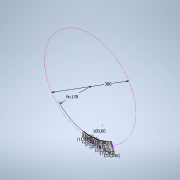
# Autodesk Inventor part: keywell_support-back
Saved by Autodesk Inventor 2020.1 (Build 241239000, 239)
## iProperties
Created: 2019-06-30
Part Number: keywell_support-back
Material: Acier inoxydable
Document SubType Name: Modeling
Designer: Thibault
Density: 8 g/cm^3
Appearance: Semi-poli
Mass: 13.686 g
Surface Area: 39.9351 cm^2
Volume: 1.71076 cm^3
kws_bp_anchor_dist1: 13,236 mm
kws_bp_anchor_dist2: 19,377 mm
kws_bp_anchor_dist3: 20,152 mm
kws_bp_anchor_dist4: 20,681 mm
kws_bp_anchor_dist5: 20,957 mm
kws_bp_anchor_dist6: 20,990 mm
kws_bp_anchor_dist7: 11,748 mm
Author: Thibault
Autodesk Inventor part; units mm, degrees
ref_plane "YZ Plane" through (0, 0, 0) normal (1, 0, 0) x (0, 1, 0)
ref_plane "XZ Plane" through (0, 0, 0) normal (0, 1, 0) x (-1, 0, 0)
ref_plane "XY Plane" through (0, 0, 0) normal (0, 0, 1) x (1, 0, 0)
sketch "Anchor (screw side)" plane through (0, 0, 0) normal (0, 0, 1) x (1, 0, 0)
  circle A0 centre (93.7216, 50.3096) radius 1.05
  line L0 (91.2716, 51.3596) -> (88.1716, 51.3596)
  line L1 (88.1716, 51.3596) -> (88.1716, 49.2596)
  line L2 (88.1716, 49.2596) -> (91.2716, 49.2596)
  line L3 (91.2716, 49.2596) -> (91.2716, 51.3596)
  line L4 (99.2716, 51.3596) -> (96.1716, 51.3596)
  line L5 (96.1716, 51.3596) -> (96.1716, 49.2596)
  line L6 (96.1716, 49.2596) -> (99.2716, 49.2596)
  line L7 (99.2716, 49.2596) -> (99.2716, 51.3596)
  line L8 (91.2716, 51.3596) -> (96.1716, 49.2596) construction
  line L9 (96.1716, 51.3596) -> (91.2716, 49.2596) construction
  line L10 (86.1716, 53.3596) -> (101.2716, 53.3596) construction
  line L11 (101.2716, 53.3596) -> (101.2716, 47.2596) construction
  line L12 (101.2716, 47.2596) -> (86.1716, 47.2596) construction
  line L13 (86.1716, 47.2596) -> (86.1716, 53.3596) construction
  point P0 (103.5798, 50.1132)
  dimension "d27" = 2.1
  dimension "d28" = 3.1
  dimension "d29" = 2.1
  dimension "d32_1" = 4.9
  dimension "d34" = 2
  dimension "d35" = 2
  dimension "d36" = 2
  dimension "d37" = 2
  measures "d27" diameter of A0
  measures "d28" distance of L2.end L1.end
  measures "d29" distance of L1.end L0.end
  measures "d32_1" distance between parallel lines of L5 L3
  measures "d34" distance between parallel lines of L0 L10
  measures "d35" distance between parallel lines of L12 L2
  measures "d36" distance between parallel lines of L11 L7
  measures "d37" distance between parallel lines of L13 L1
sketch "Anchor (nut side)" plane through (0, 0, 0) normal (0, 0, 1) x (1, 0, 0)
  line L0 (10, 0) -> (8.55, 0)
  line L1 (8.55, 0) -> (8.55, -2)
  line L2 (8.55, -2) -> (9.35, -2)
  line L3 (9.35, -2) -> (9.35, -4)
  line L4 (5.65, -4) -> (5.65, -2)
  line L5 (5.65, -2) -> (6.45, -2)
  line L6 (6.45, -2) -> (6.45, 0)
  line L7 (6.45, 0) -> (5, 0)
  line L8 (2, 0) -> (2, 2)
  line L9 (2, 0) -> (3, 0) construction
  line L10 (2, 2) -> (5, 2)
  line L11 (5, 2) -> (5, 0)
  line L12 (10, 0) -> (10, 2)
  line L13 (10, 2) -> (13, 2)
  line L14 (13, 2) -> (13, 0)
  line L15 (0, 0) -> (2, 0)
  line L16 (13, 0) -> (15, 0)
  line L17 (5.65, -4) -> (6.45, -4)
  line L18 (9.35, -4) -> (8.55, -4)
  line L19 (6.45, -4) -> (6.45, -6.25)
  line L20 (8.55, -4) -> (8.55, -6.25)
  line L21 (6.7, -6.5) -> (7.5, -6.5)
  arc A0 (6.45, -6.25) -> (6.7, -6.5) centre (6.7, -6.25) ccw
  arc A1 (8.3, -6.5) -> (8.55, -6.25) centre (8.3, -6.25) ccw
  line L22 (7.5, -6.5) -> (8.3, -6.5)
  line L23 (7.5, -3.8983) -> (7.5, -9.959) construction
  point P0 (9.1321, -0.6227)
  point P1 (6.45, -6.5)
  point P2 (8.55, -6.5)
  dimension "d3" = 2
  dimension "d7" = 5
  dimension "d10" = 1.45
  dimension "d11" = 2
  dimension "d12" = 0.8
  dimension "d13" = 2
  dimension "d14" = 0.8
  dimension "d15" = 2.1
  dimension "d18" = 2
  dimension "d19" = 0.8
  dimension "d20" = 0.8
  dimension "d21" = 2.5
  dimension "d22" = 2.5
  dimension "d23" = 2.1
  dimension "d38" = 2
  dimension "d39" = 0.25
  dimension "d120" = 3
  measures "d3" distance of point (0, 0) L8.start
  measures "d7" distance of L7.end L0.start
  measures "d10" distance of L0.start L0.end
  measures "d11" distance of L0.end L1.end
  measures "d12" distance of L1.end L2.end
  measures "d13" distance of L2.end L3.end
  measures "d14" distance of L4.end L5.end
  measures "d15" distance of L6.end L0.end
  measures "d18" distance of L14.end point (15, 0)
  measures "d19" distance of L4.start L17.end
  measures "d20" distance of L3.end L18.end
  measures "d21" distance of L17.end point (6.45, -6.5)
  measures "d22" distance of L18.end point (8.55, -6.5)
  measures "d23" distance of L17.end L18.end
  measures "d38" distance of the line from the sketch origin of L10
  measures "d39" radius of A0
  measures "d120" distance of L8.end L10.end
sketch "Screwless anchor (male)" plane through (0, 0, 0) normal (0, 0, 1) x (1, 0, 0)
  line L0 (2, 0) -> (2, 2)
  line L1 (2, 0) -> (3, 0) construction
  line L2 (2, 2) -> (5, 2)
  line L3 (5, 2) -> (5, 0)
  line L4 (10, 0) -> (10, 2)
  line L5 (10, 2) -> (13, 2)
  line L6 (13, 2) -> (13, 0)
  line L7 (0, 0) -> (2, 0)
  line L8 (13, 0) -> (15, 0)
  line L9 (5, 0) -> (10, 0)
  point P0 (9.1321, -0.6227)
  dimension "d81" = 2
  dimension "d83" = 5
  dimension "d92" = 2
  dimension "d100" = 2
  dimension "d119" = 3
  measures "d81" distance of L7.start L0.start
  measures "d83" distance of L3.end L4.start
  measures "d92" distance of L6.end L8.end
  measures "d100" distance between parallel lines of L7 L2
  measures "d119" distance of L0.end L2.end
sketch "Screwless anchor (female)" plane through (0, 0, 0) normal (0, 0, 1) x (1, 0, 0)
  line L0 (91.7814, 51.7592) -> (88.6814, 51.7592)
  line L1 (88.6814, 51.7592) -> (88.6814, 49.6592)
  line L2 (88.6814, 49.6592) -> (91.7814, 49.6592)
  line L3 (91.7814, 49.6592) -> (91.7814, 51.7592)
  line L4 (99.7814, 51.7592) -> (96.6814, 51.7592)
  line L5 (96.6814, 51.7592) -> (96.6814, 49.6592)
  line L6 (96.6814, 49.6592) -> (99.7814, 49.6592)
  line L7 (99.7814, 49.6592) -> (99.7814, 51.7592)
  line L8 (86.6814, 53.7592) -> (101.7814, 53.7592) construction
  line L9 (101.7814, 53.7592) -> (101.7814, 47.6592) construction
  line L10 (101.7814, 47.6592) -> (86.6814, 47.6592) construction
  line L11 (86.6814, 47.6592) -> (86.6814, 53.7592) construction
  point P0 (103.5798, 50.1132)
  dimension "d106" = 3.1
  dimension "d107" = 2.1
  dimension "d108" = 3.1
  dimension "d109" = 4.9
  dimension "d110" = 2
  dimension "d111" = 2
  dimension "d112" = 2
  dimension "d113" = 2
  measures "d106" distance of L2.end L1.end
  measures "d107" distance of L1.end L0.end
  measures "d108" distance of L6.end L5.end
  measures "d109" distance between parallel lines of L5 L3
  measures "d110" distance between parallel lines of L0 L8
  measures "d111" distance between parallel lines of L10 L2
  measures "d112" distance between parallel lines of L9 L7
  measures "d113" distance between parallel lines of L11 L1
sketch "Anchor" plane through (0, 0, 0) normal (0, 0, 1) x (1, 0, 0)
  line L0 (-55.5458, -124.6418) -> (-44.4458, -138.5418) construction
  line L1 (-44.4458, -124.6418) -> (-55.5458, -138.5418) construction
  line L2 (-49.9958, -129.7424) -> (-49.9958, -133.4154) construction
  circle A0 centre (-49.9958, -123.5918) radius 1.05
  line L3 (-52.4458, -122.5418) -> (-55.5458, -122.5418)
  line L4 (-55.5458, -122.5418) -> (-55.5458, -124.6418)
  line L5 (-55.5458, -124.6418) -> (-52.4458, -124.6418)
  line L6 (-52.4458, -124.6418) -> (-52.4458, -122.5418)
  line L7 (-44.4458, -122.5418) -> (-47.5458, -122.5418)
  line L8 (-47.5458, -122.5418) -> (-47.5458, -124.6418)
  line L9 (-47.5458, -124.6418) -> (-44.4458, -124.6418)
  line L10 (-44.4458, -124.6418) -> (-44.4458, -122.5418)
  line L11 (-52.4458, -122.5418) -> (-47.5458, -124.6418) construction
  line L12 (-47.5458, -122.5418) -> (-52.4458, -124.6418) construction
  line L13 (-57.5458, -120.5418) -> (-42.4458, -120.5418) construction
  line L14 (-42.4458, -120.5418) -> (-42.4458, -126.6418) construction
  line L15 (-42.4458, -126.6418) -> (-57.5458, -126.6418) construction
  line L16 (-57.5458, -126.6418) -> (-57.5458, -120.5418) construction
  circle A1 centre (-49.9958, -139.5918) radius 1.05
  line L17 (-52.4458, -138.5418) -> (-55.5458, -138.5418)
  line L18 (-55.5458, -138.5418) -> (-55.5458, -140.6418)
  line L19 (-55.5458, -140.6418) -> (-52.4458, -140.6418)
  line L20 (-52.4458, -140.6418) -> (-52.4458, -138.5418)
  line L21 (-44.4458, -138.5418) -> (-47.5458, -138.5418)
  line L22 (-47.5458, -138.5418) -> (-47.5458, -140.6418)
  line L23 (-47.5458, -140.6418) -> (-44.4458, -140.6418)
  line L24 (-44.4458, -140.6418) -> (-44.4458, -138.5418)
  line L25 (-52.4458, -138.5418) -> (-47.5458, -140.6418) construction
  line L26 (-47.5458, -138.5418) -> (-52.4458, -140.6418) construction
  line L27 (-57.5458, -136.5418) -> (-42.4458, -136.5418) construction
  line L28 (-42.4458, -136.5418) -> (-42.4458, -142.6418) construction
  line L29 (-42.4458, -142.6418) -> (-57.5458, -142.6418) construction
  line L30 (-57.5458, -142.6418) -> (-57.5458, -136.5418) construction
  point P0 (-66.8969, -206.6558)
  point P1 (-49.9958, -123.5918)
  dimension "d161" = 13.9
sketch "Esquisse2" plane through (0, 0, 0) normal (0, 0, 1) x (1, 0, 0)
  circle A0 centre (0, 0) radius 190 construction
  arc A1 (-29.0684, -175.6104) -> (87.3783, -155.0775) centre (0, 0) ccw
  line L0 (-31.0925, -195.4005) -> (-29.0684, -175.6104)
  line L1 (49.6599, -108.9569) -> (49.6599, -114.726) construction
  line L2 (96.0489, -172.9818) -> (96.0489, -198.8453)
  line L3 (-31.0925, -195.4005) -> (-31.0925, -198.8453)
  line L4 (30.9281, -182.0636) -> (33.2072, -181.6617) construction
  line L5 (87.3783, -155.0775) -> (96.0489, -172.9818)
  line L6 (-26.8444, -198.8453) -> (-31.0925, -198.8453)
  line L7 (-11.8444, -198.8453) -> (-5.8545, -198.8453)
  line L8 (9.1455, -198.8453) -> (15.1026, -198.8453)
  line L9 (30.1026, -198.8453) -> (35.7836, -198.8453)
  line L10 (50.7836, -198.8453) -> (55.9358, -198.8453)
  line L11 (70.9358, -198.8453) -> (75.313, -198.8453)
  line L12 (90.313, -198.8453) -> (96.0489, -198.8453)
  line L13 (28.843, -182.3134) -> (16.3622, -194.9882) construction
  line L14 (30.1635, -193.3346) -> (15.0417, -183.967) construction
  line L15 (24.4388, -188.4308) -> (20.7919, -188.8677) construction
  circle A2 centre (30.5458, -187.6991) radius 1.05
  line L16 (31.2969, -185.1416) -> (30.9281, -182.0636)
  line L17 (30.9281, -182.0636) -> (28.843, -182.3134)
  line L18 (28.843, -182.3134) -> (29.2118, -185.3914)
  line L19 (29.2118, -185.3914) -> (31.2969, -185.1416)
  line L20 (32.2486, -193.0848) -> (31.8798, -190.0068)
  line L21 (31.8798, -190.0068) -> (29.7947, -190.2566)
  line L22 (29.7947, -190.2566) -> (30.1635, -193.3346)
  line L23 (30.1635, -193.3346) -> (32.2486, -193.0848)
  line L24 (31.2969, -185.1416) -> (29.7947, -190.2566) construction
  line L25 (31.8798, -190.0068) -> (29.2118, -185.3914) construction
  line L26 (32.676, -179.8399) -> (34.4723, -194.8327) construction
  line L27 (34.4723, -194.8327) -> (28.4156, -195.5583) construction
  line L28 (28.4156, -195.5583) -> (26.6193, -180.5655) construction
  line L29 (26.6193, -180.5655) -> (32.676, -179.8399) construction
  circle A3 centre (14.6594, -189.6025) radius 1.05
  line L30 (15.4105, -187.045) -> (15.0417, -183.967)
  line L31 (15.0417, -183.967) -> (12.9566, -184.2168)
  line L32 (12.9566, -184.2168) -> (13.3254, -187.2948)
  line L33 (13.3254, -187.2948) -> (15.4105, -187.045)
  line L34 (16.3622, -194.9882) -> (15.9934, -191.9102)
  line L35 (15.9934, -191.9102) -> (13.9083, -192.16)
  line L36 (13.9083, -192.16) -> (14.2771, -195.238)
  line L37 (14.2771, -195.238) -> (16.3622, -194.9882)
  line L38 (15.4105, -187.045) -> (13.9083, -192.16) construction
  line L39 (15.9934, -191.9102) -> (13.3254, -187.2948) construction
  line L40 (16.7896, -181.7433) -> (18.5859, -196.736) construction
  line L41 (18.5859, -196.736) -> (12.5292, -197.4617) construction
  line L42 (12.5292, -197.4617) -> (10.7329, -182.4689) construction
  line L43 (10.7329, -182.4689) -> (16.7896, -181.7433) construction
  line L44 (86.6491, -162.9786) -> (78.9769, -179.0272) construction
  line L45 (91.4871, -172.9688) -> (74.1389, -169.0371) construction
  line L46 (84.4775, -170.1969) -> (81.1717, -171.7978) construction
  circle A4 centre (90.0132, -167.5161) radius 1.05
  line L47 (89.8903, -164.8534) -> (88.5392, -162.0633)
  line L48 (88.5392, -162.0633) -> (86.6491, -162.9786)
  line L49 (86.6491, -162.9786) -> (88.0003, -165.7687)
  line L50 (88.0003, -165.7687) -> (89.8903, -164.8534)
  line L51 (93.3772, -172.0535) -> (92.026, -169.2635)
  line L52 (92.026, -169.2635) -> (90.136, -170.1788)
  line L53 (90.136, -170.1788) -> (91.4871, -172.9688)
  line L54 (91.4871, -172.9688) -> (93.3772, -172.0535)
  line L55 (89.8903, -164.8534) -> (90.136, -170.1788) construction
  line L56 (92.026, -169.2635) -> (88.0003, -165.7687) construction
  line L57 (89.4675, -159.3916) -> (96.0489, -172.9818) construction
  line L58 (96.0489, -172.9818) -> (90.5588, -175.6405) construction
  line L59 (90.5588, -175.6405) -> (83.9774, -162.0503) construction
  line L60 (83.9774, -162.0503) -> (89.4675, -159.3916) construction
  circle A5 centre (75.6129, -174.4898) radius 1.05
  line L61 (75.4901, -171.8271) -> (74.1389, -169.0371)
  line L62 (74.1389, -169.0371) -> (72.2489, -169.9524)
  line L63 (72.2489, -169.9524) -> (73.6, -172.7424)
  line L64 (73.6, -172.7424) -> (75.4901, -171.8271)
  line L65 (78.9769, -179.0272) -> (77.6258, -176.2372)
  line L66 (77.6258, -176.2372) -> (75.7357, -177.1525)
  line L67 (75.7357, -177.1525) -> (77.0869, -179.9425)
  line L68 (77.0869, -179.9425) -> (78.9769, -179.0272)
  line L69 (75.4901, -171.8271) -> (75.7357, -177.1525) construction
  line L70 (77.6258, -176.2372) -> (73.6, -172.7424) construction
  line L71 (75.0672, -166.3653) -> (81.6487, -179.9555) construction
  line L72 (81.6487, -179.9555) -> (76.1586, -182.6143) construction
  line L73 (76.1586, -182.6143) -> (69.5771, -169.024) construction
  line L74 (69.5771, -169.024) -> (75.0672, -166.3653) construction
  line L75 (-5.2561, -195.6029) -> (8.5472, -184.3829) construction
  line L76 (-5.3523, -184.5033) -> (8.6433, -195.4825) construction
  line L77 (-0.2038, -190.0089) -> (3.4691, -189.9771) construction
  circle A6 centre (-6.3542, -190.0622) radius 1.05
  line L78 (-7.3829, -192.5212) -> (-7.3561, -195.621)
  line L79 (-7.3561, -195.621) -> (-5.2561, -195.6029)
  line L80 (-5.2561, -195.6029) -> (-5.283, -192.503)
  line L81 (-5.283, -192.503) -> (-7.3829, -192.5212)
  line L82 (-7.4522, -184.5215) -> (-7.4253, -187.6213)
  line L83 (-7.4253, -187.6213) -> (-5.3254, -187.6032)
  line L84 (-5.3254, -187.6032) -> (-5.3523, -184.5033)
  line L85 (-5.3523, -184.5033) -> (-7.4522, -184.5215)
  line L86 (-7.3829, -192.5212) -> (-5.3254, -187.6032) construction
  line L87 (-7.4253, -187.6213) -> (-5.283, -192.503) construction
  line L88 (-9.3387, -197.6383) -> (-9.4694, -182.5389) construction
  line L89 (-9.4694, -182.5389) -> (-3.3697, -182.486) construction
  line L90 (-3.3697, -182.486) -> (-3.2389, -197.5855) construction
  line L91 (-3.2389, -197.5855) -> (-9.3387, -197.6383) construction
  circle A7 centre (9.6452, -189.9236) radius 1.05
  line L92 (8.6165, -192.3826) -> (8.6433, -195.4825)
  line L93 (8.6433, -195.4825) -> (10.7433, -195.4643)
  line L94 (10.7433, -195.4643) -> (10.7164, -192.3644)
  line L95 (10.7164, -192.3644) -> (8.6165, -192.3826)
  line L96 (8.5472, -184.3829) -> (8.5741, -187.4828)
  line L97 (8.5741, -187.4828) -> (10.674, -187.4646)
  line L98 (10.674, -187.4646) -> (10.6471, -184.3647)
  line L99 (10.6471, -184.3647) -> (8.5472, -184.3829)
  line L100 (8.6165, -192.3826) -> (10.674, -187.4646) construction
  line L101 (8.5741, -187.4828) -> (10.7164, -192.3644) construction
  line L102 (6.6607, -197.4997) -> (6.53, -182.4003) construction
  line L103 (6.53, -182.4003) -> (12.6297, -182.3475) construction
  line L104 (12.6297, -182.3475) -> (12.7605, -197.4469) construction
  line L105 (12.7605, -197.4469) -> (6.6607, -197.4997) construction
  line L106 (-26.8103, -193.8281) -> (-11.853, -184.1999) construction
  line L107 (-25.6809, -182.7857) -> (-12.9824, -195.2423) construction
  line L108 (-21.1714, -188.8258) -> (-17.5175, -189.1995) construction
  circle A8 centre (-27.2901, -188.2) radius 1.05
  line L109 (-28.5839, -190.5305) -> (-28.8994, -193.6144)
  line L110 (-28.8994, -193.6144) -> (-26.8103, -193.8281)
  line L111 (-26.8103, -193.8281) -> (-26.4948, -190.7441)
  line L112 (-26.4948, -190.7441) -> (-28.5839, -190.5305)
  line L113 (-27.77, -182.572) -> (-28.0854, -185.6559)
  line L114 (-28.0854, -185.6559) -> (-25.9963, -185.8696)
  line L115 (-25.9963, -185.8696) -> (-25.6809, -182.7857)
  line L116 (-25.6809, -182.7857) -> (-27.77, -182.572)
  line L117 (-28.5839, -190.5305) -> (-25.9963, -185.8696) construction
  line L118 (-28.0854, -185.6559) -> (-26.4948, -190.7441) construction
  line L119 (-31.0925, -195.4005) -> (-29.5561, -180.3789) construction
  line L120 (-29.5561, -180.3789) -> (-23.4878, -180.9995) construction
  line L121 (-23.4878, -180.9995) -> (-25.0241, -196.0212) construction
  line L122 (-25.0241, -196.0212) -> (-31.0925, -195.4005) construction
  circle A9 centre (-11.3732, -189.828) radius 1.05
  line L123 (-12.667, -192.1584) -> (-12.9824, -195.2423)
  line L124 (-12.9824, -195.2423) -> (-10.8933, -195.456)
  line L125 (-10.8933, -195.456) -> (-10.5779, -192.3721)
  line L126 (-10.5779, -192.3721) -> (-12.667, -192.1584)
  line L127 (-11.853, -184.1999) -> (-12.1684, -187.2838)
  line L128 (-12.1684, -187.2838) -> (-10.0793, -187.4975)
  line L129 (-10.0793, -187.4975) -> (-9.7639, -184.4136)
  line L130 (-9.7639, -184.4136) -> (-11.853, -184.1999)
  line L131 (-12.667, -192.1584) -> (-10.0793, -187.4975) construction
  line L132 (-12.1684, -187.2838) -> (-10.5779, -192.3721) construction
  line L133 (-15.1755, -197.0284) -> (-13.6391, -182.0068) construction
  line L134 (-13.6391, -182.0068) -> (-7.5708, -182.6275) construction
  line L135 (-7.5708, -182.6275) -> (-9.1072, -197.6491) construction
  line L136 (-9.1072, -197.6491) -> (-15.1755, -197.0284) construction
  line L137 (48.7865, -178.0168) -> (37.7806, -191.9915) construction
  line L138 (51.3152, -188.8249) -> (35.252, -181.1833) construction
  line L139 (45.0843, -184.5828) -> (41.5079, -185.4196) construction
  circle A10 centre (51.0732, -183.1817) radius 1.05
  line L140 (51.5375, -180.5569) -> (50.8313, -177.5384)
  line L141 (50.8313, -177.5384) -> (48.7865, -178.0168)
  line L142 (48.7865, -178.0168) -> (49.4927, -181.0353)
  line L143 (49.4927, -181.0353) -> (51.5375, -180.5569)
  line L144 (53.3599, -188.3465) -> (52.6537, -185.3281)
  line L145 (52.6537, -185.3281) -> (50.6089, -185.8065)
  line L146 (50.6089, -185.8065) -> (51.3152, -188.8249)
  line L147 (51.3152, -188.8249) -> (53.3599, -188.3465)
  line L148 (51.5375, -180.5569) -> (50.6089, -185.8065) construction
  line L149 (52.6537, -185.3281) -> (49.4927, -181.0353) construction
  line L150 (52.3231, -175.1354) -> (55.763, -189.8383) construction
  line L151 (55.763, -189.8383) -> (49.8234, -191.228) construction
  line L152 (49.8234, -191.228) -> (46.3835, -176.525) construction
  line L153 (46.3835, -176.525) -> (52.3231, -175.1354) construction
  circle A11 centre (35.4939, -186.8266) radius 1.05
  line L154 (35.9582, -184.2018) -> (35.252, -181.1833)
  line L155 (35.252, -181.1833) -> (33.2072, -181.6617)
  line L156 (33.2072, -181.6617) -> (33.9134, -184.6802)
  line L157 (33.9134, -184.6802) -> (35.9582, -184.2018)
  line L158 (37.7806, -191.9915) -> (37.0744, -188.973)
  line L159 (37.0744, -188.973) -> (35.0297, -189.4514)
  line L160 (35.0297, -189.4514) -> (35.7359, -192.4699)
  line L161 (35.7359, -192.4699) -> (37.7806, -191.9915)
  line L162 (35.9582, -184.2018) -> (35.0297, -189.4514) construction
  line L163 (37.0744, -188.973) -> (33.9134, -184.6802) construction
  line L164 (36.7438, -178.7803) -> (40.1837, -193.4833) construction
  line L165 (40.1837, -193.4833) -> (34.2441, -194.8729) construction
  line L166 (34.2441, -194.8729) -> (30.8042, -180.1699) construction
  line L167 (30.8042, -180.1699) -> (36.7438, -178.7803) construction
  line L168 (68.134, -171.5455) -> (58.7376, -186.6494) construction
  line L169 (71.84, -182.0086) -> (55.0316, -176.1864) construction
  line L170 (65.179, -178.48) -> (61.7168, -179.7063) construction
  circle A12 centre (70.9767, -176.4265) radius 1.05
  line L171 (71.1485, -173.7665) -> (70.1135, -170.8444)
  line L172 (70.1135, -170.8444) -> (68.134, -171.5455)
  line L173 (68.134, -171.5455) -> (69.169, -174.4676)
  line L174 (69.169, -174.4676) -> (71.1485, -173.7665)
  line L175 (73.8194, -181.3075) -> (72.7844, -178.3853)
  line L176 (72.7844, -178.3853) -> (70.8049, -179.0865)
  line L177 (70.8049, -179.0865) -> (71.84, -182.0086)
  line L178 (71.84, -182.0086) -> (73.8194, -181.3075)
  line L179 (71.1485, -173.7665) -> (70.8049, -179.0865) construction
  line L180 (72.7844, -178.3853) -> (69.169, -174.4676) construction
  line L181 (71.331, -168.2914) -> (76.3724, -182.5249) construction
  line L182 (76.3724, -182.5249) -> (70.6225, -184.5616) construction
  line L183 (70.6225, -184.5616) -> (65.581, -170.328) construction
  line L184 (65.581, -170.328) -> (71.331, -168.2914) construction
  circle A13 centre (55.8948, -181.7685) radius 1.05
  line L185 (56.0666, -179.1085) -> (55.0316, -176.1864)
  line L186 (55.0316, -176.1864) -> (53.0521, -176.8875)
  line L187 (53.0521, -176.8875) -> (54.0871, -179.8096)
  line L188 (54.0871, -179.8096) -> (56.0666, -179.1085)
  line L189 (58.7376, -186.6494) -> (57.7026, -183.7273)
  line L190 (57.7026, -183.7273) -> (55.7231, -184.4284)
  line L191 (55.7231, -184.4284) -> (56.7581, -187.3505)
  line L192 (56.7581, -187.3505) -> (58.7376, -186.6494)
  line L193 (56.0666, -179.1085) -> (55.7231, -184.4284) construction
  line L194 (57.7026, -183.7273) -> (54.0871, -179.8096) construction
  line L195 (56.2491, -173.6334) -> (61.2905, -187.8669) construction
  line L196 (61.2905, -187.8669) -> (55.5406, -189.9035) construction
  line L197 (55.5406, -189.9035) -> (50.4991, -175.67) construction
  line L198 (50.4991, -175.67) -> (56.2491, -173.6334) construction
  line L199 (-21.8444, -198.8453) -> (-20.3944, -198.8453)
  line L200 (-20.3944, -198.8453) -> (-20.3944, -196.8453)
  line L201 (-20.3944, -196.8453) -> (-21.1944, -196.8453)
  line L202 (-21.1944, -196.8453) -> (-21.1944, -194.8453)
  line L203 (-17.4944, -194.8453) -> (-17.4944, -196.8453)
  line L204 (-17.4944, -196.8453) -> (-18.2944, -196.8453)
  line L205 (-18.2944, -196.8453) -> (-18.2944, -198.8453)
  line L206 (-18.2944, -198.8453) -> (-16.8444, -198.8453)
  line L207 (-13.8444, -198.8453) -> (-13.8444, -200.8453)
  line L208 (-13.8444, -198.8453) -> (-14.8444, -198.8453) construction
  line L209 (-13.8444, -200.8453) -> (-16.8444, -200.8453)
  line L210 (-16.8444, -200.8453) -> (-16.8444, -198.8453)
  line L211 (-21.8444, -198.8453) -> (-21.8444, -200.8453)
  line L212 (-21.8444, -200.8453) -> (-24.8444, -200.8453)
  line L213 (-24.8444, -200.8453) -> (-24.8444, -198.8453)
  line L214 (-11.8444, -198.8453) -> (-13.8444, -198.8453)
  line L215 (-24.8444, -198.8453) -> (-26.8444, -198.8453)
  line L216 (-17.4944, -194.8453) -> (-18.2944, -194.8453)
  line L217 (-21.1944, -194.8453) -> (-20.3944, -194.8453)
  line L218 (-18.2944, -194.8453) -> (-18.2944, -192.5953)
  line L219 (-20.3944, -194.8453) -> (-20.3944, -192.5953)
  line L220 (-18.5444, -192.3453) -> (-19.3444, -192.3453)
  arc A14 (-18.2944, -192.5953) -> (-18.5444, -192.3453) centre (-18.5444, -192.5953) ccw
  arc A15 (-20.1444, -192.3453) -> (-20.3944, -192.5953) centre (-20.1444, -192.5953) ccw
  line L221 (-19.3444, -192.3453) -> (-20.1444, -192.3453)
  line L222 (-19.3444, -194.9471) -> (-19.3444, -188.8863) construction
  line L223 (-0.8545, -198.8453) -> (0.5955, -198.8453)
  line L224 (0.5955, -198.8453) -> (0.5955, -196.8453)
  line L225 (0.5955, -196.8453) -> (-0.2045, -196.8453)
  line L226 (-0.2045, -196.8453) -> (-0.2045, -194.8453)
  line L227 (3.4955, -194.8453) -> (3.4955, -196.8453)
  line L228 (3.4955, -196.8453) -> (2.6955, -196.8453)
  line L229 (2.6955, -196.8453) -> (2.6955, -198.8453)
  line L230 (2.6955, -198.8453) -> (4.1455, -198.8453)
  line L231 (7.1455, -198.8453) -> (7.1455, -200.8453)
  line L232 (7.1455, -198.8453) -> (6.1455, -198.8453) construction
  line L233 (7.1455, -200.8453) -> (4.1455, -200.8453)
  line L234 (4.1455, -200.8453) -> (4.1455, -198.8453)
  line L235 (-0.8545, -198.8453) -> (-0.8545, -200.8453)
  line L236 (-0.8545, -200.8453) -> (-3.8545, -200.8453)
  line L237 (-3.8545, -200.8453) -> (-3.8545, -198.8453)
  line L238 (9.1455, -198.8453) -> (7.1455, -198.8453)
  line L239 (-3.8545, -198.8453) -> (-5.8545, -198.8453)
  line L240 (3.4955, -194.8453) -> (2.6955, -194.8453)
  line L241 (-0.2045, -194.8453) -> (0.5955, -194.8453)
  line L242 (2.6955, -194.8453) -> (2.6955, -192.5953)
  line L243 (0.5955, -194.8453) -> (0.5955, -192.5953)
  line L244 (2.4455, -192.3453) -> (1.6455, -192.3453)
  arc A16 (2.6955, -192.5953) -> (2.4455, -192.3453) centre (2.4455, -192.5953) ccw
  arc A17 (0.8455, -192.3453) -> (0.5955, -192.5953) centre (0.8455, -192.5953) ccw
  line L245 (1.6455, -192.3453) -> (0.8455, -192.3453)
  line L246 (1.6455, -194.9471) -> (1.6455, -188.8863) construction
  line L247 (20.1026, -198.8453) -> (21.5526, -198.8453)
  line L248 (21.5526, -198.8453) -> (21.5526, -196.8453)
  line L249 (21.5526, -196.8453) -> (20.7526, -196.8453)
  line L250 (20.7526, -196.8453) -> (20.7526, -194.8453)
  line L251 (24.4526, -194.8453) -> (24.4526, -196.8453)
  line L252 (24.4526, -196.8453) -> (23.6526, -196.8453)
  line L253 (23.6526, -196.8453) -> (23.6526, -198.8453)
  line L254 (23.6526, -198.8453) -> (25.1026, -198.8453)
  line L255 (28.1026, -198.8453) -> (28.1026, -200.8453)
  line L256 (28.1026, -198.8453) -> (27.1026, -198.8453) construction
  line L257 (28.1026, -200.8453) -> (25.1026, -200.8453)
  line L258 (25.1026, -200.8453) -> (25.1026, -198.8453)
  line L259 (20.1026, -198.8453) -> (20.1026, -200.8453)
  line L260 (20.1026, -200.8453) -> (17.1026, -200.8453)
  line L261 (17.1026, -200.8453) -> (17.1026, -198.8453)
  line L262 (30.1026, -198.8453) -> (28.1026, -198.8453)
  line L263 (17.1026, -198.8453) -> (15.1026, -198.8453)
  line L264 (24.4526, -194.8453) -> (23.6526, -194.8453)
  line L265 (20.7526, -194.8453) -> (21.5526, -194.8453)
  line L266 (23.6526, -194.8453) -> (23.6526, -192.5953)
  line L267 (21.5526, -194.8453) -> (21.5526, -192.5953)
  line L268 (23.4026, -192.3453) -> (22.6026, -192.3453)
  arc A18 (23.6526, -192.5953) -> (23.4026, -192.3453) centre (23.4026, -192.5953) ccw
  arc A19 (21.8026, -192.3453) -> (21.5526, -192.5953) centre (21.8026, -192.5953) ccw
  line L269 (22.6026, -192.3453) -> (21.8026, -192.3453)
  line L270 (22.6026, -194.9471) -> (22.6026, -188.8863) construction
  line L271 (40.7836, -198.8453) -> (42.2336, -198.8453)
  line L272 (42.2336, -198.8453) -> (42.2336, -196.8453)
  line L273 (42.2336, -196.8453) -> (41.4336, -196.8453)
  line L274 (41.4336, -196.8453) -> (41.4336, -194.8453)
  line L275 (45.1336, -194.8453) -> (45.1336, -196.8453)
  line L276 (45.1336, -196.8453) -> (44.3336, -196.8453)
  line L277 (44.3336, -196.8453) -> (44.3336, -198.8453)
  line L278 (44.3336, -198.8453) -> (45.7836, -198.8453)
  line L279 (48.7836, -198.8453) -> (48.7836, -200.8453)
  line L280 (48.7836, -198.8453) -> (47.7836, -198.8453) construction
  line L281 (48.7836, -200.8453) -> (45.7836, -200.8453)
  line L282 (45.7836, -200.8453) -> (45.7836, -198.8453)
  line L283 (40.7836, -198.8453) -> (40.7836, -200.8453)
  line L284 (40.7836, -200.8453) -> (37.7836, -200.8453)
  line L285 (37.7836, -200.8453) -> (37.7836, -198.8453)
  line L286 (50.7836, -198.8453) -> (48.7836, -198.8453)
  line L287 (37.7836, -198.8453) -> (35.7836, -198.8453)
  line L288 (45.1336, -194.8453) -> (44.3336, -194.8453)
  line L289 (41.4336, -194.8453) -> (42.2336, -194.8453)
  line L290 (44.3336, -194.8453) -> (44.3336, -192.5953)
  line L291 (42.2336, -194.8453) -> (42.2336, -192.5953)
  line L292 (44.0836, -192.3453) -> (43.2836, -192.3453)
  arc A20 (44.3336, -192.5953) -> (44.0836, -192.3453) centre (44.0836, -192.5953) ccw
  arc A21 (42.4836, -192.3453) -> (42.2336, -192.5953) centre (42.4836, -192.5953) ccw
  line L293 (43.2836, -192.3453) -> (42.4836, -192.3453)
  line L294 (43.2836, -194.9471) -> (43.2836, -188.8863) construction
  line L295 (60.9358, -198.8453) -> (62.3858, -198.8453)
  line L296 (62.3858, -198.8453) -> (62.3858, -196.8453)
  line L297 (62.3858, -196.8453) -> (61.5858, -196.8453)
  line L298 (61.5858, -196.8453) -> (61.5858, -194.8453)
  line L299 (65.2858, -194.8453) -> (65.2858, -196.8453)
  line L300 (65.2858, -196.8453) -> (64.4858, -196.8453)
  line L301 (64.4858, -196.8453) -> (64.4858, -198.8453)
  line L302 (64.4858, -198.8453) -> (65.9358, -198.8453)
  line L303 (68.9358, -198.8453) -> (68.9358, -200.8453)
  line L304 (68.9358, -198.8453) -> (67.9358, -198.8453) construction
  line L305 (68.9358, -200.8453) -> (65.9358, -200.8453)
  line L306 (65.9358, -200.8453) -> (65.9358, -198.8453)
  line L307 (60.9358, -198.8453) -> (60.9358, -200.8453)
  line L308 (60.9358, -200.8453) -> (57.9358, -200.8453)
  line L309 (57.9358, -200.8453) -> (57.9358, -198.8453)
  line L310 (70.9358, -198.8453) -> (68.9358, -198.8453)
  line L311 (57.9358, -198.8453) -> (55.9358, -198.8453)
  line L312 (65.2858, -194.8453) -> (64.4858, -194.8453)
  line L313 (61.5858, -194.8453) -> (62.3858, -194.8453)
  line L314 (64.4858, -194.8453) -> (64.4858, -192.5953)
  line L315 (62.3858, -194.8453) -> (62.3858, -192.5953)
  line L316 (64.2358, -192.3453) -> (63.4358, -192.3453)
  arc A22 (64.4858, -192.5953) -> (64.2358, -192.3453) centre (64.2358, -192.5953) ccw
  arc A23 (62.6358, -192.3453) -> (62.3858, -192.5953) centre (62.6358, -192.5953) ccw
  line L317 (63.4358, -192.3453) -> (62.6358, -192.3453)
  line L318 (63.4358, -194.9471) -> (63.4358, -188.8863) construction
  line L319 (80.313, -198.8453) -> (81.763, -198.8453)
  line L320 (81.763, -198.8453) -> (81.763, -196.8453)
  line L321 (81.763, -196.8453) -> (80.963, -196.8453)
  line L322 (80.963, -196.8453) -> (80.963, -194.8453)
  line L323 (84.663, -194.8453) -> (84.663, -196.8453)
  line L324 (84.663, -196.8453) -> (83.863, -196.8453)
  line L325 (83.863, -196.8453) -> (83.863, -198.8453)
  line L326 (83.863, -198.8453) -> (85.313, -198.8453)
  line L327 (88.313, -198.8453) -> (88.313, -200.8453)
  line L328 (88.313, -198.8453) -> (87.313, -198.8453) construction
  line L329 (88.313, -200.8453) -> (85.313, -200.8453)
  line L330 (85.313, -200.8453) -> (85.313, -198.8453)
  line L331 (80.313, -198.8453) -> (80.313, -200.8453)
  line L332 (80.313, -200.8453) -> (77.313, -200.8453)
  line L333 (77.313, -200.8453) -> (77.313, -198.8453)
  line L334 (90.313, -198.8453) -> (88.313, -198.8453)
  line L335 (77.313, -198.8453) -> (75.313, -198.8453)
  line L336 (84.663, -194.8453) -> (83.863, -194.8453)
  line L337 (80.963, -194.8453) -> (81.763, -194.8453)
  line L338 (83.863, -194.8453) -> (83.863, -192.5953)
  line L339 (81.763, -194.8453) -> (81.763, -192.5953)
  line L340 (83.613, -192.3453) -> (82.813, -192.3453)
  arc A24 (83.863, -192.5953) -> (83.613, -192.3453) centre (83.613, -192.5953) ccw
  arc A25 (82.013, -192.3453) -> (81.763, -192.5953) centre (82.013, -192.5953) ccw
  line L341 (82.813, -192.3453) -> (82.013, -192.3453)
  line L342 (82.813, -194.9471) -> (82.813, -188.8863) construction
  point P0 (1.6455, -189.9929)
  point P1 (-19.3316, -189.014)
  point P2 (43.2836, -185.0041)
  point P3 (63.4358, -179.0975)
  point P4 (22.6026, -188.6508)
  point P5 (82.813, -171.0029)
  point P6 (-19.3316, -189.014)
  point P7 (1.6455, -189.9929)
  point P8 (22.6026, -188.6508)
  point P9 (63.4358, -179.0975)
  point P10 (82.813, -171.0029)
  point P11 (82.813, -171.0029)
  point P12 (63.4358, -179.0975)
  point P13 (43.2836, -185.0041)
  point P14 (22.6026, -188.6508)
  point P15 (1.6455, -189.9929)
  point P16 (-19.3444, -189.0127)
  dimension "kws_bp_anchor_dist2" = 19.3773
  dimension "kws_bp_anchor_dist3" = 20.1522
  dimension "kws_bp_anchor_dist4" = 20.681
  dimension "kws_bp_anchor_dist5" = 20.9571
  dimension "kws_bp_anchor_dist6" = 20.99
  dimension "radius" = 380
  dimension "d73" = 178
  dimension "d163" = 21
  dimension "d164" = 21
  dimension "d165" = 21
  dimension "d166" = 21
  dimension "d167" = 21
  dimension "d170" = 80
  dimension "kws_bp_anchor_dist1" = 13.236
  dimension "kws_bp_anchor_dist7" = 11.748
  constraints: 26 end point, 8 point on circle, 7 horizontal, 3 vertical, 2 centre point, 1 coincident, 49 other
  measures "radius" diameter of A0
  measures "d73" radius of A1
  measures "d163" distance of A0.start A0.end
  measures "d164" distance of point (22.603, -188.651) point (43.284, -185.004)
  measures "d165" distance of point (43.284, -185.004) point (63.436, -179.097)
  measures "d166" distance of point (63.436, -179.097) point (82.813, -171.003)
  measures "d167" distance of A0.start point (22.603, -188.651)
  measures "d170" angle of L4 L1
extrude "Base" add sketch "Esquisse2" along normal blind 2
sketch "Esquisse5" plane through (0, 0, 2) normal (0, 0, 1) x (1, 0, 0)
  line L0 (50.2059, -108.6494) -> (185.6965, -108.6494)
  line L1 (185.6965, -108.6494) -> (185.6965, -257.0945)
  line L2 (50.2059, -108.6494) -> (76.3724, -182.5249)
  line L3 (76.3724, -182.5249) -> (76.3724, -257.0945)
  line L4 (76.3724, -257.0945) -> (185.6965, -257.0945)
  line L5 (70.1135, -170.8444) -> (71.1485, -173.7665) projected
  line L6 (73.8194, -181.3075) -> (71.84, -182.0086) projected
  point P0 (0, 0)
  dimension "d171" = 2
  dimension "d172" = 2
  constraints: 10 end point, 2 perpendicular, 1 horizontal, 1 parallel, 1 vertical
  measures "d171" distance between parallel lines of L5 L2
  measures "d172" distance from line of L2.end L6
extrude "Front: substract" [suppressed]
sketch "Esquisse7" plane through (0, 0, 2) normal (0, 0, 1) x (1, 0, 0)
  line L0 (74.4872, -183.1927) -> (56.3302, -131.9301)
  line L1 (72.7854, -178.388) -> (73.2029, -179.5666)
  line L2 (-107.1306, -265.4008) -> (-95.5548, -119.8506)
  line L3 (-95.5548, -119.8506) -> (56.3302, -131.9301)
  line L4 (74.4872, -183.1927) -> (74.4872, -265.4008)
  line L5 (74.4872, -265.4008) -> (-107.1306, -265.4008)
  line L6 (73.6, -172.7424) -> (72.2489, -169.9524) projected
  line L7 (70.1135, -170.8444) -> (71.1485, -173.7665) projected
  line L8 (73.8194, -181.3075) -> (71.84, -182.0086) projected
  point P0 (0, 0)
  dimension "d175" = 2
  constraints: 12 end point, 2 collinear, 2 perpendicular, 1 vertical
  measures "d175" distance from line of L0.start L8
extrude "Front r6: substract" [suppressed]
derived "shared_parameters.ipt"
sketch "Esquisse9" plane through (0, 0, 2) normal (0, 0, 1) x (1, 0, 0)
  line L0 (90.313, -175.7596) -> (173.7897, -135.3336)
  line L1 (93.3772, -172.0535) -> (91.4871, -172.9688) projected
  line L2 (90.313, -175.7596) -> (90.313, -265.0884)
  line L3 (88.313, -200.8453) -> (88.313, -198.8453) projected
  line L4 (173.7897, -135.3336) -> (173.7897, -265.0884)
  line L5 (173.7897, -265.0884) -> (90.313, -265.0884)
  point P0 (0, 0)
  dimension "d192" = 2
  dimension "d193" = 2
  constraints: 9 end point, 2 vertical, 1 parallel, 1 perpendicular
  measures "d192" distance between parallel lines of L0 L1
  measures "d193" distance between parallel lines of L2 L3
extrude "Gain de place" [suppressed]
equation "\"esd\" = 0.1"
